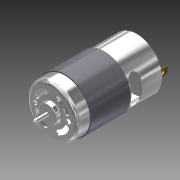
# Autodesk Inventor part: RS-395
Saved by Autodesk Inventor 2015 SP1 (Build 190203100, 203)
## iProperties
Category: Motors
Company: Autodesk, Inc.
Shininess: 64.0
Length Units: 11269
Angle Units: 11279
Time Units: 11290
Mass Units: 11283
Length Display Precision: 3
Angle Display Precision: 2
Compacted: True
Part Number: RS-395
Document SubType Name: Modeling
Created: 2014-12-12
Material: Steel, Mild
Project: FIRST
Catalog Web Link: http://banebots.com/pc/MOTOR-BRUSH/M5-RS395-12
Vendor: BaneBots
Density: 7.67073 g/cm^3
Description: Motor - BaneBots RS-395
Mass: 96 g
Surface Area: 100.567 cm^2
Volume: 4.74254 cm^3
Appearance: Chrome - Polished
Density: 0.0
Volumn: 0.0
Area: 0.0
PropertySet Name: Model Information
Control State: 0
Master: False
Checked Out: False
Title: Motor - BaneBots RS-550
Author: Autodesk, Inc.
Autodesk Inventor part; units mm, degrees
note: some values were not read from the file. Chosen so that the rebuilt part matches the saved one: direction of "Hole3".
sketch "Sketch1" plane through (0, 0, 0) normal (0, 0, 1) x (1, 0, 0)
  circle A0 centre (0, 0) radius 13.75
  dimension "d0" = 27.5
  constraints: 2 coincident, 1 centre point, 2 other
  measures "d0" diameter of A0
extrude "Extrusion1" add sketch "Sketch1" along normal mid plane 46.1
fillet "Fillet1" radius 2 1 edges at (-13.75, 0, 23.05)
shell "Shell1" thickness 0.62 removed faces 1 at (-0.6469, -3.772, -23.05)
sketch "Sketch2" plane through (0, 0, 23.05) normal (0, 0, 1) x (1, 0, 0)
  circle A0 centre (0, 0) radius 11.75 projected
  circle A1 centre (0, 0) radius 5
  dimension "d5" = 10
  constraints: 1 centre point, 1 coincident, 1 concentric
  measures "d5" diameter of A1
extrude "Extrusion2" add sketch "Sketch2" along normal blind 2.5 contours A1
fillet "Fillet2" radius 0.5 2 edges at (-5, 0, 23.05) (-5, 0, 25.55)
sketch "Sketch3" plane through (0, 0, 25.55) normal (0, 0, 1) x (1, 0, 0)
  circle A0 centre (0, 0) radius 4.5 projected
  circle A1 centre (0, 0) radius 1.15
  dimension "d9" = 2.3
  constraints: 1 centre point, 1 coincident, 1 concentric
  measures "d9" diameter of A1
extrude "Extrusion3" add sketch "Sketch3" along normal blind 7.6 contours A1
fillet "Fillet3" radius 1.15 1 edges at (-1.15, 0, 33.15)
sketch "Sketch4" plane through (0, 0, 23.05) normal (0, 0, 1) x (1, 0, 0)
  circle A0 centre (0, 0) radius 11.75 projected
  point P0 (9, 0)
  dimension "d13" = 9
  constraints: 1 horizontal alignment
  measures "d13" distance of point (9, 0) A0.centre
hole "Hole1" at (9, 0, 23.05) direction (0, 0, -1) diameter 2.5 depth 8 tip angle 118
mirror "Mirror1" about plane through (0, 0, 0) normal (1, 0, 0) of "Hole1"
sketch "Sketch5" plane through (0, 0, 23.05) normal (0, 0, 1) x (1, 0, 0)
  circle A0 centre (9, 0) radius 1.25 projected
  circle A1 centre (0, 0) radius 5.5 projected
  arc A2 (9.1904, 3.9415) -> (3.9678, 9.1791) centre (0, 0) ccw
  arc A3 (6.8928, 2.9562) -> (2.9759, 6.8843) centre (0, 0) ccw
  line L0 (0, 0) -> (1.9411, 7.2444) construction
  line L1 (0, 0) -> (8.3652, 2.2414) construction
  line L2 (0, 0) -> (9, 0) construction
  line L3 (0.151, 0.5634) -> (0.151, 14.7153) construction
  arc A4 (3.9678, 9.1791) -> (2.9759, 6.8843) centre (3.4719, 8.0317) ccw
  arc A5 (6.8928, 2.9562) -> (9.1904, 3.9415) centre (8.0416, 3.4488) ccw
  point P0 (7.2444, 1.9411)
  dimension "d21" = 15
  dimension "d22" = 15
  dimension "d23" = 10
  dimension "d24" = 7.5
  constraints: 9 point on circle, 8 end point, 4 centre point, 4 tangent, 2 coincident, 2 concentric, 2 point on line, 1 horizontal, 1 perpendicular
  measures "d21" angle of L1 L2
  measures "d22" angle of L3 L0
  measures "d23" radius of A2
  measures "d24" radius of A3
extrude "Extrusion4" cut sketch "Sketch5" against normal blind 10 contours A5 A3 A4 A2
pattern_circular "Circular Pattern1" count 4 over 360 about axis through (0, 0, 0) along (0, 0, 1) of "Extrusion4"
ref_plane "Work Plane1" through (0, 0, -21.3) normal (0, 0, -1) x (-1, 0, 0)
sketch "Sketch6" plane through (0, 0, -21.3) normal (0, 0, -1) x (-1, 0, 0)
  circle A0 centre (0, 0) radius 13.13 projected
extrude "Extrusion5" add sketch "Sketch6" against normal blind 0.62
sketch "Sketch7" plane through (0, 0, -21.3) normal (0, 0, -1) x (-1, 0, 0)
  circle A0 centre (0, 0) radius 13.13 projected
  circle A1 centre (0, 0) radius 10
  dimension "d33" = 20
  constraints: 1 centre point, 1 coincident, 1 concentric
  measures "d33" diameter of A1
extrude "Extrusion6" add sketch "Sketch7" along normal blind 0.62 contours A1
sketch "Sketch8" plane through (0, 0, -21.92) normal (0, 0, -1) x (-1, 0, 0)
  circle A0 centre (0, 0) radius 10 projected
  circle A1 centre (0, 0) radius 5.375
  dimension "d36" = 10.75
  constraints: 1 centre point, 1 coincident, 1 concentric
  measures "d36" diameter of A1
extrude "Extrusion7" add sketch "Sketch8" along normal blind 3 contours A1
sketch "Sketch9" plane through (0, 0, -24.92) normal (0, 0, -1) x (-1, 0, 0)
  circle A0 centre (0, 0) radius 5.375 projected
  circle A1 centre (0, 0) radius 3.45
  dimension "d39" = 6.9
  constraints: 1 centre point, 1 coincident, 1 concentric
  measures "d39" diameter of A1
extrude "Extrusion8" cut sketch "Sketch9" against normal blind 0.8 contours A1
sketch "Sketch10" plane through (0, 0, -24.12) normal (0, 0, -1) x (-1, 0, 0)
  circle A0 centre (0, 0) radius 3.45 projected
  circle A1 centre (0, 0) radius 1.6
  dimension "d42" = 3.2
  constraints: 1 centre point, 1 coincident, 1 concentric
  measures "d42" diameter of A1
extrude "Extrusion9" add sketch "Sketch10" along normal blind 1 contours A1
sketch "Sketch11" plane through (0, 0, -21.92) normal (0, 0, -1) x (-1, 0, 0)
  circle A0 centre (0, 0) radius 5.375 projected
  circle A1 centre (0, 0) radius 10 projected
  arc A2 (8.4307, 3.15) -> (3.15, 8.4307) centre (0, 0) ccw
  arc A3 (5.1066, 3.15) -> (3.15, 5.1066) centre (0, 0) ccw
  line L0 (3.15, 8.4307) -> (3.15, 5.1066)
  line L1 (5.1066, 3.15) -> (8.4307, 3.15)
  dimension "d45" = 3.15
  dimension "d46" = 3.15
  dimension "d47" = 9
  dimension "d48" = 6
  constraints: 4 end point, 4 point on circle, 2 centre point, 2 coincident, 2 concentric, 1 perpendicular, 1 vertical
  measures "d45" distance from line of L0 A3.centre
  measures "d46" distance from line of A0.centre L1
  measures "d47" radius of A2
  measures "d48" radius of A3
extrude "Extrusion10" cut sketch "Sketch11" against normal blind 1 contours L1 A3 L0 A2
pattern_circular "Circular Pattern2" count 4 over 360 about axis through (0, 0, 0) along (0, 0, 1) of "Extrusion10"
sketch "Sketch12" plane through (0, 0, -21.3) normal (0, 0, -1) x (-1, 0, 0)
  circle A0 centre (0, 0) radius 10 projected
  circle A1 centre (0, 0) radius 13.13 projected
  line L0 (-11.5, 1.9) -> (-11, 1.9)
  line L1 (-11, 1.9) -> (-11, -1.9)
  line L2 (-11, -1.9) -> (-11.5, -1.9)
  line L3 (-11.5, -1.9) -> (-11.5, 1.9)
  line L4 (0, 0) -> (-16.9017, 0) construction
  point P0 (-11, 0)
  dimension "d54" = 0.5
  dimension "d55" = 3.8
  dimension "d56" = 11
  constraints: 10 end point, 2 parallel, 2 perpendicular, 1 horizontal, 1 midpoint, 1 point on line
  measures "d54" distance of L1.end L2.end
  measures "d55" distance of L2.end L0.start
  measures "d56" distance from line of L1 A0.centre
extrude "Extrusion11" add sketch "Sketch12" along normal blind 7.2 contours L0 L1 L2 L3
chamfer "Chamfer1" distance 1 angle 45 2 edges at (11.25, 1.9, -28.5) (11.25, -1.9, -28.5)
sketch "Sketch13" plane through (11.5, 0, 0) normal (1, 0, 0) x (0, 0, -1)
  line L0 (28.5, -0.9) -> (28.5, 0.9) projected
  line L1 (25.5, 0) -> (27.5, 1.9) construction
  line L2 (25.5, 0) -> (27.5, -1.9) construction
  dimension "d79" = 3
  constraints: 4 end point, 1 equal length
  measures "d79" distance from line of L0 L1.start
hole "Hole3" at (11.5, 0, -25.5) direction (-1, 0, 0) diameter 2 end up to surface
mirror "Mirror2" about plane through (0, 0, 0) normal (1, 0, 0) of "Extrusion11", "Chamfer1", "Hole3"
ref_plane "Work Plane2" through (18, 0, 0) normal (1, 0, 0) x (0, 1, 0)
sketch "Sketch14" plane through (18, 0, 0) normal (1, 0, 0) x (0, 1, 0)
  arc A0 (-4.5554, -6.4) -> (-4.5554, -12.3) centre (-4.5554, -9.35) ccw
  arc A1 (5.2946, -12.3) -> (5.2946, -6.4) centre (5.2946, -9.35) ccw
  line L0 (-4.5554, -6.4) -> (5.2946, -6.4)
  line L1 (-4.5554, -12.3) -> (5.2946, -12.3)
  line L2 (13.75, -23.05) -> (-13.75, -23.05) projected
  line L3 (0, -23.05) -> (0, 22.6064) construction
  dimension "d70" = 10.75
  dimension "d71" = 5.9
  dimension "d72" = 9.85
  constraints: 6 end point, 4 point on circle, 4 tangent, 2 centre point, 1 equal radius, 1 horizontal, 1 horizontal alignment, 1 midpoint, 1 parallel, 1 perpendicular
  measures "d70" distance between parallel lines of L2 L1
  measures "d71" distance between parallel lines of L0 L1
  measures "d72" distance of A1.centre A0.centre
extrude "Extrusion12" cut sketch "Sketch14" against normal through all
ref_plane "Work Plane3" through (0, 0, 21.05) normal (0, 0, -1) x (-1, 0, 0)
ref_plane "Work Plane4" through (0, 0, 16.05) normal (0, 0, 1) x (1, 0, 0)
sketch "Sketch16" plane through (0, 0, 16.05) normal (0, 0, 1) x (1, 0, 0)
  circle A0 centre (0, 0) radius 13.75 projected
  circle A1 centre (0, 0) radius 14.4
  dimension "d88" = 0.65
  constraints: 1 centre point, 1 coincident
  measures "d88" radial gap between concentric circles of A1 A0
extrude "Extrusion14" add sketch "Sketch16" against normal blind 21.5
body "Solid1"
